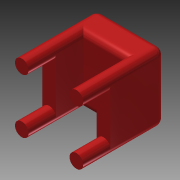
# Autodesk Inventor part: Short Brace Prototype Mk1
Saved by Autodesk Inventor 2015 (Build 190159000, 159)
## iProperties
Created: 2016-11-23
Part Number: Short Brace Prototype Mk1
Material: Generic
Document SubType Name: Modeling
Designer: Markus
Density: 1 g/cm^3
Appearance: Light Red
Author: Markus
Autodesk Inventor part; units mm, degrees
ref_plane "YZ Plane" through (0, 0, 0) normal (1, 0, 0) x (0, 1, 0)
ref_plane "XZ Plane" through (0, 0, 0) normal (0, 1, 0) x (-1, 0, 0)
ref_plane "XY Plane" through (0, 0, 0) normal (0, 0, 1) x (1, 0, 0)
sketch "Sketch1" plane through (0, 0, 0) normal (0, 0, 1) x (1, 0, 0)
  line L0 (0, 0) -> (15.875, 0)
  line L1 (15.875, 0) -> (15.875, 15.875)
  line L2 (15.875, 15.875) -> (0, 15.875)
  line L3 (0, 15.875) -> (0, 0)
  dimension "d0" = 15.875
  dimension "d1" = 15.875
  constraints: 8 end point, 2 parallel, 1 horizontal, 1 perpendicular
  measures "d0" distance of L0.start L0.end
  measures "d1" distance of L2.end L0.start
extrude "Extrusion1" add sketch "Sketch1" along normal blind 6.35
sketch "Sketch2" plane through (0, 0, 6.35) normal (0, 0, 1) x (1, 0, 0)
  line L0 (0, 0) -> (15.875, 0) projected
  line L1 (0, 15.875) -> (3.175, 15.875)
  line L2 (3.175, 15.875) -> (3.175, 0)
  line L3 (3.175, 0) -> (0, 0)
  line L4 (0, 0) -> (0, 15.875)
  line L5 (15.875, 0) -> (12.7, 0)
  line L6 (12.7, 0) -> (12.7, 15.875)
  line L7 (12.7, 15.875) -> (15.875, 15.875)
  line L8 (15.875, 15.875) -> (15.875, 0)
  point P0 (0, 15.875)
  point P1 (0, 7.9375)
  dimension "d4" = 3.175
  constraints: 16 end point, 4 parallel, 2 horizontal, 2 perpendicular, 2 point on line, 1 collinear, 1 horizontal alignment, 1 midpoint, 1 vertical alignment
  measures "d4" distance of L2.end L3.end
extrude "Extrusion2" add sketch "Sketch2" along normal blind 6.35
sketch "Sketch3" plane through (0, 0, 12.7) normal (0, 0, 1) x (1, 0, 0)
  line L0 (0, 15.875) -> (0, 0) projected
  line L1 (0, 0) -> (3.175, 0) projected
  line L2 (3.175, 0) -> (3.175, 15.875) projected
  line L3 (3.175, 15.875) -> (0, 15.875) projected
  line L4 (15.875, 0) -> (15.875, 15.875) projected
  line L5 (15.875, 15.875) -> (12.7, 15.875) projected
  line L6 (12.7, 15.875) -> (12.7, 0) projected
  line L7 (12.7, 0) -> (15.875, 0) projected
  circle A0 centre (1.5875, 14.2875) radius 1.5875
  circle A1 centre (14.2875, 14.2875) radius 1.5875
  circle A2 centre (14.2875, 1.5875) radius 1.5875
  circle A3 centre (1.5875, 1.5875) radius 1.5875
  constraints: 12 tangent, 4 centre point
extrude "Extrusion3" add sketch "Sketch3" along normal blind 6.35 contours A0 | A3 | A2 | A1
fillet "Fillet1" radius 1.5875 6 edges at (3.175, 15.875, 9.525) (12.7, 15.875, 9.525) (3.175, 0, 9.525) (12.7, 0, 9.525) (7.9375, 0, 6.35) (7.9375, 15.875, 6.35)
fillet "Fillet2" radius 1.5875 8 edges at (0, 15.875, 6.35) (15.875, 15.875, 6.35) (0, 0, 6.35) (15.875, 0, 6.35) (7.9375, 0, 0) (15.875, 7.9375, 0) (7.9375, 15.875, 0) (0, 7.9375, 0)
sketch "Sketch4" plane through (1.5875, 15.875, 4.7625) normal (0, 1, 0) x (1, 0, 0)
  line L0 (0, 0) -> (0, 3.175) projected
  line L1 (12.7, 0) -> (0, 0) projected
  line L2 (12.7, 3.175) -> (12.7, 0) projected
  line L3 (0, 3.175) -> (12.7, 3.175) projected
  line L4 (1.7487, 3.2269) -> (9.4749, 3.2269) construction
  line L5 (9.4749, 3.2269) -> (9.4749, 0.0505) construction
  line L6 (9.4749, 0.0505) -> (1.7487, 0.0505) construction
  line L7 (1.7487, 0.0505) -> (1.7487, 3.2269) construction
  point P0 (-1.5875, 4.7625)
  constraints: 2 other
body "Solid1"
